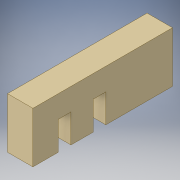
# Autodesk Inventor part: LargeSideHook
Saved by Autodesk Inventor 2016 (Build 200138000, 138)
## iProperties
Created: 2016-06-15
Part Number: LargeSideHook
Material: Generic
Document SubType Name: Modeling
Designer: cutrones
Density: 1 g/cm^3
Appearance: Beige
Author: cutrones
Autodesk Inventor part; units mm, degrees
ref_plane "YZ Plane" through (0, 0, 0) normal (1, 0, 0) x (0, 1, 0)
ref_plane "XZ Plane" through (0, 0, 0) normal (0, 1, 0) x (-1, 0, 0)
ref_plane "XY Plane" through (0, 0, 0) normal (0, 0, 1) x (1, 0, 0)
sketch "Sketch1" plane through (0, 0, 0) normal (0, 0, 1) x (1, 0, 0)
  line L0 (0, 0) -> (50.8, 0)
  line L1 (50.8, 0) -> (50.8, 101.6)
  line L2 (50.8, 101.6) -> (0, 101.6)
  line L3 (0, 101.6) -> (0, 0)
  dimension "d0" = 50.8
  dimension "d1" = 101.6
  constraints: 8 end point, 2 parallel, 1 horizontal, 1 perpendicular
  measures "d0" distance of L2.end L1.end
  measures "d1" distance of L1.end L0.end
extrude "Extrusion1" add sketch "Sketch1" along normal blind 279.4
sketch "Sketch2" plane through (50.8, 0, 0) normal (1, 0, 0) x (0, 0, -1)
  line L0 (0, 0) -> (-279.4, 0) projected
  line L1 (-228.6, 0) -> (-203.2, 0)
  line L2 (-203.2, 0) -> (-203.2, 57.15)
  line L3 (-203.2, 57.15) -> (-228.6, 57.15)
  line L4 (-228.6, 57.15) -> (-228.6, 0)
  line L5 (-279.4, 0) -> (-279.4, 101.6) projected
  line L6 (-158.75, 0) -> (-133.35, 0)
  line L7 (-133.35, 0) -> (-133.35, 57.15)
  line L8 (-133.35, 57.15) -> (-158.75, 57.15)
  line L9 (-158.75, 57.15) -> (-158.75, 0)
  dimension "d4" = 25.4
  dimension "d5" = 57.15
  dimension "d6" = 50.8
  dimension "d7" = 25.4
  dimension "d8" = 44.45
  constraints: 16 end point, 4 parallel, 2 horizontal, 2 perpendicular, 2 point on line
  measures "d4" distance of L3.end L2.end
  measures "d5" distance of L2.end L1.end
  measures "d6" distance between parallel lines of L5 L4
  measures "d7" distance of L8.end L7.end
  measures "d8" distance between parallel lines of L2 L9
extrude "Extrusion2" cut sketch "Sketch2" against normal blind 266.7
body "Solid1"
